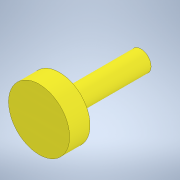
# Autodesk Inventor part: clutch02-releaseMechanism
Saved by Autodesk Inventor 2021 (Build 250183000, 183)
## iProperties
Created: 2020-07-03
Part Number: clutch02-releaseMechanism
Material: PET Plastic
Document SubType Name: Modeling
Designer: robst
Density: 1.541 g/cm^3
Appearance: Canary
Author: robst
Autodesk Inventor part; units mm, degrees
ref_plane "YZ Plane" through (0, 0, 0) normal (1, 0, 0) x (0, 1, 0)
ref_plane "XZ Plane" through (0, 0, 0) normal (0, 1, 0) x (-1, 0, 0)
ref_plane "XY Plane" through (0, 0, 0) normal (0, 0, 1) x (1, 0, 0)
ref_plane "Work Plane1" through (0, 0, 0) normal (0, 0, 1) x (1, 0, 0)
sketch "Sketch1" plane through (0, 0, 0) normal (0, 0, 1) x (1, 0, 0)
  circle A0 centre (0, 0) radius 12.7
  dimension "d0" = 25.4
  constraints: 1 centre point, 1 coincident
  measures "d0" diameter of A0
extrude "Extrusion1" add sketch "Sketch1" against normal blind 50.8
sketch "Sketch2" plane through (0, 0, 0) normal (0, 0, 1) x (1, 0, 0)
  circle A0 centre (0, 0) radius 12.7
  constraints: 1 centre point, 1 coincident
extrude "Extrusion2" add sketch "Sketch2" along normal blind 50.8
sketch "Sketch4" plane through (0, 0, 50.8) normal (0, 0, 1) x (1, 0, 0)
  circle A0 centre (0, 0) radius 38.1
  dimension "d6" = 76.2
  constraints: 1 centre point, 1 coincident
  measures "d6" diameter of A0
extrude "Extrusion3" add sketch "Sketch4" along normal blind 25.4
ref_plane "Work Plane2" through (175.2488, -178.5172, -25.4) normal (0, 0, 1) x (0.350341, -0.9366222, 0)
sketch "Sketch5" plane through (175.2488, -178.5172, -25.4) normal (0, 0, 1) x (0.350341, -0.9366222, 0)
  circle A0 centre (-228.6, -101.6) radius 12.7 construction
  line L0 (-228.6, -114.3) -> (-228.6, -88.9) construction
  line L1 (-225.425, -107.95) -> (-231.775, -107.95)
  line L2 (-231.775, -107.95) -> (-231.775, -120.65)
  line L3 (-231.775, -120.65) -> (-225.425, -120.65)
  line L4 (-225.425, -120.65) -> (-225.425, -107.95)
  line L5 (-225.425, -107.95) -> (-231.775, -120.65) construction
  line L6 (-231.775, -107.95) -> (-225.425, -120.65) construction
  dimension "d9" = 6.35
  dimension "d10" = 12.7
  constraints: 14 end point, 2 midpoint, 2 parallel, 2 point on circle, 1 horizontal, 1 perpendicular, 1 vertical
  measures "d9" distance of L2.end L3.end
  measures "d10" distance of L3.end L1.start
extrude "Extrusion4" add sketch "Sketch5" along normal blind 25.4
body "Solid1"
